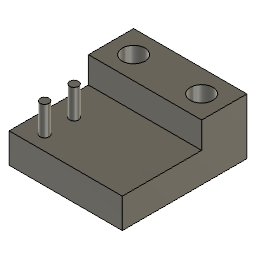
EndtasterHalter (Autodesk Fusion 360 design; units mm, degrees)
part number: 2025-12-04-22-20-04-428
Autodesk Fusion 360 part; units mm, degrees
note: some values were not read from the file. Set by a fixed rule: which sketch regions a step uses.
sketch "Skizze1" plane through (0, 0, 0) normal (0, 1, 0) x (1, 0, 0)
  line L0 (0, 0) -> (25, 0)
  line L1 (25, 0) -> (25, -15)
  line L2 (25, -15) -> (0, -15)
  line L3 (0, -15) -> (0, 0)
  line L4 (25, -15) -> (20, -15)
  line L5 (20, -15) -> (20, -10)
  line L6 (20, -10) -> (25, -10)
  line L7 (25, -10) -> (25, -15)
  circle A0 centre (20, -10) radius 2.5
  line L8 (0, -15) -> (5, -15)
  line L9 (5, -15) -> (5, -10)
  line L10 (5, -10) -> (0, -10)
  line L11 (0, -10) -> (0, -15)
  circle A1 centre (5, -10) radius 2.5
  dimension "d1" = 25
  dimension "d2" = 15
  dimension "d3" = 5
  dimension "d4" = 5
  dimension "d5" = 5
  dimension "d7" = 5
  dimension "d8" = 5
  dimension "d9" = 5
  constraint horizontal L0
  constraint vertical L1
  constraint horizontal L2
  constraint vertical L3
  constraint coincident L0.start L3.end
  constraint horizontal L4
  constraint vertical L5
  constraint horizontal L6
  constraint vertical L7
  constraint coincident L5.end L6.start
  constraint horizontal L8
  constraint vertical L9
  constraint horizontal L10
  constraint vertical L11
  constraint coincident L9.end L10.start
  measures "d1" distance of L0.start L0.end
  measures "d2" distance of L0.start L2.end
  measures "d3" distance of L1.end L4.end
  measures "d4" distance of L1.end L6.end
  measures "d5" diameter of A0
  measures "d7" distance of L2.end L8.end
  measures "d8" distance of L2.end L10.end
  measures "d9" diameter of A1
extrude "Extrusion1" add sketch "Skizze1" along normal blind 8 contours L0 L1 L2 L3 L5 L6 A0 L9 L10 A1 | L2 L3 L8 L9 L10 L11 A1 | L1 L2 L4 L5 L6 L7 A0
move_body "Verschieben1" bodies 1 to x (1, 0, 0) y (0, 0, -1) z (0, 1, 0) at (0, 0, 8)
extrude "Extrusion2" add 1 faces at (8.3333, 0, 5.3333) along direction (0, -1, 0) blind 12.5
sketch "Skizze2" plane through (0, 0, 8) normal (0, 0, 1) x (-1, 0, 0)
  circle A0 centre (-5, -10) radius 2.5
  circle A1 centre (-20, -10) radius 2.5
  line L0 (0, -15) -> (0, 12.5)
  line L1 (0, 12.5) -> (-25, 12.5)
  line L2 (-25, 12.5) -> (-25, -15)
  line L3 (-25, -15) -> (0, -15)
  line L4 (0, 12.5) -> (-4.6, 12.5)
  line L5 (-4.6, 12.5) -> (-4.6, -15) construction
  line L6 (-4.6, 12.5) -> (-4.6, -0.5) construction
  line L7 (-4.6, -0.5) -> (0, -0.5) construction
  line L8 (-4.6, 12.5) -> (-4.6, 9.25)
  circle A2 centre (-4.6, 9.25) radius 1
  line L9 (-4.6, 9.25) -> (-4.6, 2.75)
  circle A3 centre (-4.6, 2.75) radius 1
  dimension "d14" = 4.6
  dimension "d15" = 3.25
  dimension "d16" = 2
  dimension "d17" = 6.5
  dimension "d18" = 2
  constraint coincident L0.end L1.start
  constraint perpendicular L0 L4
  constraint coincident L3 L5.end
  constraint perpendicular L3 L5
  constraint coincident L5 L6.end
  constraint coincident L0 L7.end
  constraint perpendicular L0 L7
  constraint perpendicular L4 L8
  constraint coincident L8.end A2.centre
  constraint parallel L5 L9
  constraint coincident L9.end A3.centre
  measures "d14" distance of L0.end L4.end
  measures "d15" distance of L4.end L8.end
  measures "d16" diameter of A2
  measures "d17" distance of L8.end L9.end
  measures "d18" diameter of A3
extrude "Extrusion3" add sketch "Skizze2" along normal blind 5 contours L8 A2 L9 | L8 A2 L9 | A3
sketch "Skizze3" plane through (0, 0, 8) normal (0, 0, 1) x (-1, 0, 0)
  circle A0 centre (-4.6, 9.25) radius 1
  circle A1 centre (-4.6, 2.75) radius 1
  circle A2 centre (-5, -10) radius 2.5
  circle A3 centre (-20, -10) radius 2.5
  line L0 (0, -15) -> (0, 12.5)
  line L1 (0, 12.5) -> (-25, 12.5)
  line L2 (-25, 12.5) -> (-25, -15)
  line L3 (-25, -15) -> (0, -15)
move_body "Verschieben2" bodies 1 to x (1, 0, 0) y (0, 1, 0) z (0, 0, 1) at (0, 12, 0)
sketch "Skizze4" plane through (0, 0, 8) normal (0, 0, 1) x (-1, 0, 0)
  circle A0 centre (-4.6, -2.75) radius 1
  circle A1 centre (-4.6, -9.25) radius 1
  circle A2 centre (-5, -22) radius 2.5
  circle A3 centre (-20, -22) radius 2.5
  line L0 (0, -27) -> (0, 0.5)
  line L1 (0, 0.5) -> (-25, 0.5)
  line L2 (-25, 0.5) -> (-25, -27)
  line L3 (-25, -27) -> (0, -27)
  line L4 (0, -17) -> (-25, -17)
  constraint coincident L0 L4.start
  constraint coincident L2 L4.end
  constraint perpendicular L2 L4
extrude "Extrusion4" add sketch "Skizze4" along normal blind 4 contours L0 L2 L3 L4
extrude "Extrusion5" add 1 faces at (14.8146, 26.1458, 12) along direction (0, 0, 1) blind 0.4
extrude "Extrusion6" cut 1 faces at (18.5296, 8.5337, 8) along direction (0, 0, -1) blind 1.4
